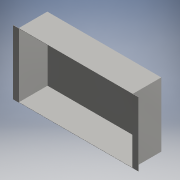
# Autodesk Inventor part: coolant tray
Saved by Autodesk Inventor 2018 (Build 220112000, 112)
## iProperties
Part Number: coolant tray
Material: Steel
Document SubType Name: Modeling
Designer: P446509
Density: 7.85 g/cm^3
Appearance: Steel
Author: P446509
Autodesk Inventor part; units mm, degrees
ref_plane "YZ Plane" through (0, 0, 0) normal (1, 0, 0) x (0, 1, 0)
ref_plane "XZ Plane" through (0, 0, 0) normal (0, 1, 0) x (-1, 0, 0)
ref_plane "XY Plane" through (0, 0, 0) normal (0, 0, 1) x (1, 0, 0)
sketch "Sketch1" plane through (0, 0, 0) normal (0, 0, 1) x (1, 0, 0)
  line L0 (0, 0) -> (7980, 0)
  line L1 (7980, 0) -> (7980, 4500)
  line L2 (7980, 4500) -> (0, 4500)
  line L3 (0, 4500) -> (0, 0)
  dimension "d0" = 7980
  dimension "d1" = 4500
  constraints: 8 end point, 2 parallel, 1 horizontal, 1 perpendicular
  measures "d0" distance of L2.end L1.end
  measures "d1" distance of L1.end L0.end
extrude "Extrusion1" add sketch "Sketch1" along normal blind 1.6
sketch "Sketch2" plane through (0, 0, 1.6) normal (0, 0, 1) x (1, 0, 0)
  line L0 (7980, 4500) -> (0, 4500) projected
  line L1 (0, 0) -> (7980, 0) projected
  line L2 (0, 4500) -> (7980, 4500)
  line L3 (7980, 4500) -> (7980, 0)
  line L4 (7980, 0) -> (0, 0)
  line L5 (0, 0) -> (0, 4500)
  line L6 (7964, 4484) -> (16, 4484)
  line L7 (16, 4484) -> (16, 16)
  line L8 (16, 16) -> (7964, 16)
  line L9 (7964, 16) -> (7964, 4484)
  dimension "d4" = 16
  constraints: 16 end point, 3 parallel, 1 horizontal, 1 perpendicular, 1 other
  measures "d4" distance between parallel lines of L0 L6
extrude "Extrusion2" add sketch "Sketch2" along normal blind 2000
sketch "Sketch3" plane through (0, 0, 0) normal (-1, 0, 0) x (0, 0, 1)
  line L0 (1.6, 4484) -> (2001.6, 4484) projected
  line L1 (2001.6, 4484) -> (1985.6, 4484)
  line L2 (1985.6, 4484) -> (1985.6, -16)
  line L3 (1985.6, -16) -> (2001.6, -16)
  line L4 (2001.6, -16) -> (2001.6, 4484)
  point P0 (0, 0)
  dimension "d7" = 16
  dimension "d8" = 4500
  constraints: 8 end point, 2 parallel, 1 horizontal, 1 perpendicular
  measures "d7" distance of L3.end L2.end
  measures "d8" distance of L2.end L1.end
extrude "Extrusion3" add sketch "Sketch3" along normal blind 400
sketch "Sketch4" plane through (7980, 0, 0) normal (1, 0, 0) x (0, 0, -1)
  line L0 (-2001.6, -16) -> (-2001.6, 0) projected
  line L1 (-2001.6, 0) -> (-1985.6, 0)
  line L2 (-1985.6, 0) -> (-1985.6, 4500)
  line L3 (-1985.6, 4500) -> (-2001.6, 4500)
  line L4 (-2001.6, 4500) -> (-2001.6, 0)
  point P0 (0, 0)
  dimension "d11" = 16
  dimension "d12" = 4500
  constraints: 8 end point, 2 parallel, 1 horizontal, 1 perpendicular
  measures "d11" distance of L3.end L2.end
  measures "d12" distance of L2.end L1.end
extrude "Extrusion4" add sketch "Sketch4" along normal blind 400
body "Solid1"
